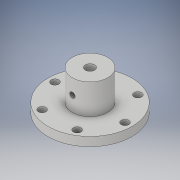
# Autodesk Inventor part: Mechanum Wheel Adapter
Saved by Autodesk Inventor 2017 (Build 210142000, 142)
## iProperties
Created: 2017-07-26
Part Number: Mechanum Wheel Adapter
Material: Generic
Document SubType Name: Modeling
Designer: User
Density: 1 g/cm^3
Appearance: Default
Author: User
Autodesk Inventor part; units mm, degrees
ref_plane "YZ Plane" through (0, 0, 0) normal (1, 0, 0) x (0, 1, 0)
ref_plane "XZ Plane" through (0, 0, 0) normal (0, 1, 0) x (-1, 0, 0)
ref_plane "XY Plane" through (0, 0, 0) normal (0, 0, 1) x (1, 0, 0)
sketch "Sketch1" plane through (0, 0, 0) normal (0, 0, 1) x (1, 0, 0)
  line L0 (0, 0) -> (0, 26.4) construction
  line L1 (3.175, 26.4) -> (3.175, 0)
  line L2 (28.4, 0) -> (28.4, 6)
  line L3 (3.175, 0) -> (28.4, 0)
  line L4 (3.175, 26.4) -> (12, 26.4)
  line L5 (12, 26.4) -> (12, 6)
  line L6 (12, 6) -> (28.4, 6)
  line L7 (12, 26.4) -> (12, -232.68) construction
  line L8 (12, 26.4) -> (12, 16.2) construction
  dimension "d0" = 26.4
  dimension "d5" = 6
  dimension "d7" = 25.225
  dimension "d11" = 8.825
  dimension "d12" = 259.08
  constraints: 18 end point, 3 vertical, 2 horizontal, 2 point on line, 1 perpendicular
  measures "d0" distance of L0.start L0.end
  measures "d5" distance of L2.start L2.end
  measures "d7" distance of L1.end L2.start
  measures "d11" distance of L1.start L4.end
  measures "d12" distance of L4.end L7.end
revolve "Revolution1" add sketch "Sketch1" angle 360 about axis through (0, 0, 0) along (0, 1, 0)
sketch "Sketch2" plane through (0, 26.4, 0) normal (0, 1, 0) x (1, 0, 0)
  circle A0 centre (0, 0) radius 12 projected
  point P0 (0, -12)
  constraints: 1 vertical alignment, 1 other
ref_plane "Work Plane1" through (0, 26.4, 12) normal (0, 0, 1) x (1, 0, 0)
sketch "Sketch3" plane through (0, 26.4, 12) normal (0, 0, 1) x (1, 0, 0)
  line L0 (-3.175, 0) -> (3.175, 0) construction
  line L1 (0, 0) -> (0, -10.2) construction
  point P0 (0, -26.4)
  dimension "d15" = 10.2
  constraints: 2 end point, 1 coincident, 1 midpoint, 1 vertical
  measures "d15" distance of L1.start L1.end
hole "Hole1" at (0, 16.2, 12) direction (0, 0, -1) diameter 3.683 depth 12 tip angle 118 thread size "10-24 UNC" class "2B" standard "ANSI Unified Screw Threads"
sketch "Sketch4" plane through (0, 6, 0) normal (0, 1, 0) x (1, 0, 0)
  line L0 (0, 0) -> (-23.75, 0) construction
  circle A0 centre (-23.75, 0) radius 2.6
  circle A1 centre (-11.875, -20.5681) radius 2.6
  circle A2 centre (11.875, -20.5681) radius 2.6
  circle A3 centre (23.75, 0) radius 2.6
  circle A4 centre (11.875, 20.5681) radius 2.6
  circle A5 centre (-11.875, 20.5681) radius 2.6
  dimension "d23" = 23.75
  dimension "d24" = 5.2
  dimension "d27" = 360
  constraints: 6 centre point, 2 end point, 1 coincident, 1 horizontal, 13 other
  measures "d23" distance of L0.start L0.end
  measures "d24" diameter of A0
extrude "Extrusion1" cut sketch "Sketch4" against normal blind 6
body "Solid1"
